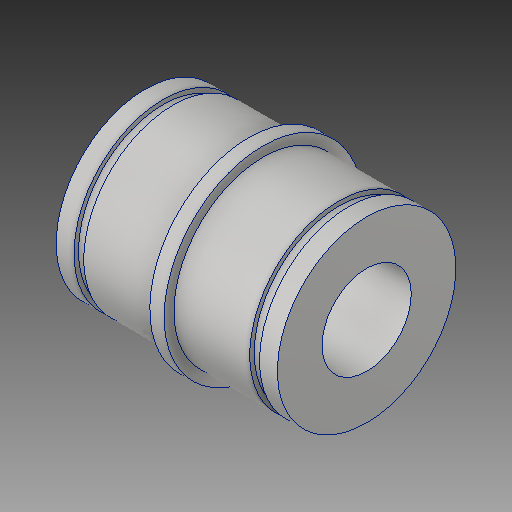
# Autodesk Inventor part: Turret Idle Pin
Saved by Autodesk Inventor 2019.4 (Build 234330000, 330)
## iProperties
Created: 2020-01-23
Part Number: Turret Idle Pin
Material: Aluminum 6061
Document SubType Name: Modeling
Designer: admin
Density: 2.7 g/cm^3
Appearance: Aluminum - Flat
Mass: 15.9101 g
Surface Area: 30.8109 cm^2
Volume: 5.89264 cm^3
Author: admin
Autodesk Inventor part; units mm, degrees
ref_plane "YZ Plane" through (0, 0, 0) normal (1, 0, 0) x (0, 1, 0)
ref_plane "XZ Plane" through (0, 0, 0) normal (0, 1, 0) x (-1, 0, 0)
ref_plane "XY Plane" through (0, 0, 0) normal (0, 0, 1) x (1, 0, 0)
sketch "Sketch1" plane through (0, 0, 0) normal (0, 0, 1) x (1, 0, 0)
  line L0 (0, 0) -> (0, 10)
  line L1 (0, 10) -> (2, 10)
  line L2 (2, 10) -> (2, 9.5)
  line L3 (2, 9.5) -> (3.1, 9.5)
  line L4 (3.1, 9.5) -> (3.1, 10)
  line L5 (3.1, 10) -> (11.6, 10)
  line L6 (11.6, 10) -> (11.6, 11.1)
  line L7 (11.6, 11.1) -> (13.2, 11.1)
  line L8 (13.2, 11.1) -> (13.2, 10)
  line L9 (13.2, 10) -> (21.7, 10)
  line L10 (21.7, 10) -> (21.7, 9.5)
  line L11 (21.7, 9.5) -> (22.8, 9.5)
  line L12 (22.8, 9.5) -> (22.8, 10)
  line L13 (22.8, 10) -> (24.8, 10)
  line L14 (24.8, 10) -> (24.8, 0)
  line L15 (24.8, 0) -> (0, 0)
  dimension "d0" = 1.1
  dimension "d1" = 2
  dimension "d2" = 0.5
  dimension "d3" = 1.1
  dimension "d4" = 1.6
  dimension "d5" = 8.5
  dimension "d6" = 1.1
  dimension "d7" = 8.5
  dimension "d8" = 2
  dimension "d9" = 10
  constraints: 32 end point, 11 perpendicular, 8 point on line, 1 vertical
  measures "d0" distance of L2.end L3.end
  measures "d1" distance of L0.end L1.end
  measures "d2" distance of L1.end L2.end
  measures "d3" distance of L5.end L6.end
  measures "d4" distance of L6.end L7.end
  measures "d5" distance of L4.end L5.end
  measures "d6" distance of L10.end L11.end
  measures "d7" distance of L8.end L9.end
  measures "d8" distance of L12.end L13.end
  measures "d9" distance between parallel lines of L15 L5
revolve "Revolution1" add sketch "Sketch1" angle 360 about axis through (24.8, 0, 0) along (-1, 0, 0)
sketch "Sketch2" plane through (24.8, 0, 0) normal (1, 0, 0) x (0, 0, -1)
  circle A0 centre (0, 0) radius 10 projected
  constraints: 1 coincident
hole "Hole1" at (24.8, 0, 0) direction (-1, 0, 0) diameter 10 end through all
body "Solid1"
